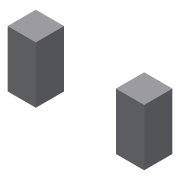
# Autodesk Inventor part: Опоры
Saved by Autodesk Inventor 2014 SP1 (Build 180222100, 222)
## iProperties
Created: 2023-10-15
Part Number: Опоры
Material: Типовые
Document SubType Name: Modeling
Designer: Konstantin
Density: 1 g/cm^3
Appearance: По умолчанию
Author: Konstantin
Autodesk Inventor part; units mm, degrees
ref_plane "YZ Plane" through (0, 0, 0) normal (1, 0, 0) x (0, 1, 0)
ref_plane "XZ Plane" through (0, 0, 0) normal (0, 1, 0) x (-1, 0, 0)
ref_plane "XY Plane" through (0, 0, 0) normal (0, 0, 1) x (1, 0, 0)
sketch "Опоры" plane through (0, 0, 0) normal (0, 1, 0) x (-1, 0, 0)
  line L0 (-14.1422, 35) -> (-24.142, 35)
  line L1 (-24.142, 35) -> (-24.142, 15)
  line L2 (-24.142, 15) -> (-14.1422, 15)
  line L3 (-14.1422, 15) -> (-14.1422, 35)
  line L4 (14.1421, 35) -> (24.1422, 35)
  line L5 (24.1422, 35) -> (24.1422, 15)
  line L6 (24.1422, 15) -> (14.1421, 15)
  line L7 (14.1421, 15) -> (14.1421, 35)
  point P0 (0, 0)
  constraints: 16 end point, 4 parallel, 2 horizontal, 2 perpendicular
extrude "Выдавливание8" add sketch "Опоры" along normal mid plane 10
